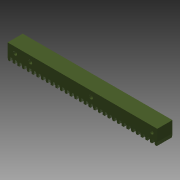
# Autodesk Inventor part: rack
Saved by Autodesk Inventor 2015 (Build 190159000, 159)
## iProperties
Created: 2015-01-14
Part Number: rack
Material: Nylon, molybdenum disulphide
Document SubType Name: Modeling
Designer: Jarod
Density: 1.13 g/cm^3
Appearance: Nylon 6
Author: Jarod
Autodesk Inventor part; units mm, degrees
ref_plane "YZ Plane" through (0, 0, 0) normal (1, 0, 0) x (0, 1, 0)
ref_plane "XZ Plane" through (0, 0, 0) normal (0, 1, 0) x (-1, 0, 0)
ref_plane "XY Plane" through (0, 0, 0) normal (0, 0, 1) x (1, 0, 0)
sketch "Sketch1" plane through (0, 0, 0) normal (1, 0, 0) x (0, 1, 0)
  line L0 (0, 0) -> (25.4, 0)
  line L1 (25.4, 0) -> (25.4, -25.4)
  line L2 (25.4, -25.4) -> (0, -25.4)
  line L3 (0, -25.4) -> (0, 0)
  dimension "d0" = 25.4
  dimension "d1" = 25.4
  constraints: 8 end point, 2 parallel, 1 horizontal, 1 perpendicular
  measures "d0" distance of L1.end L2.end
  measures "d1" distance of L0.end L1.end
extrude "Extrusion1" add sketch "Sketch1" along normal blind 254
sketch "Sketch2" plane through (0, 0, 0) normal (0, 0, 1) x (1, 0, 0)
  line L0 (0, 0) -> (0, 25.4) projected
  line L1 (0, 0) -> (254, 0) projected
  line L2 (254, 25.4) -> (254, 0) projected
  line L3 (0, 25.4) -> (254, 25.4) projected
  line L4 (0, 0) -> (0.7938, 0) construction
  line L5 (0.7938, 0) -> (0.7937, 6.35) construction
  line L6 (0.7937, 6.35) -> (0, 6.35) construction
  line L7 (0, 6.35) -> (0, 0) construction
  line L8 (0.7937, 6.35) -> (3.9687, 6.35) construction
  line L9 (3.9687, 6.35) -> (3.9687, 0) construction
  line L10 (3.9687, 0) -> (0.7938, 0) construction
  line L11 (0.7938, 0) -> (0.7937, 6.35) construction
  line L12 (3.9687, 6.35) -> (4.7625, 6.35) construction
  line L13 (4.7625, 6.35) -> (4.7625, 0) construction
  line L14 (4.7625, 0) -> (3.9687, 0) construction
  line L15 (3.9687, 0) -> (3.9687, 6.35) construction
  line L16 (0, 6.35) -> (0.7938, 0)
  line L17 (0.7938, 0) -> (3.9687, 0)
  line L18 (4.7625, 6.35) -> (7.9375, 6.35) construction
  line L19 (7.9375, 6.35) -> (7.9375, 0) construction
  line L20 (7.9375, 0) -> (4.7625, 0) construction
  line L21 (4.7625, 0) -> (4.7625, 6.35) construction
  line L22 (3.9687, 0) -> (4.7625, 6.35)
  line L23 (4.7625, 6.35) -> (7.9375, 6.35)
  line L24 (7.9375, 6.35) -> (7.9375, 0)
  line L25 (0, 6.35) -> (0, 0)
  line L26 (0, 0) -> (0.7938, 0)
  line L27 (3.9687, 0) -> (7.9375, 0)
  dimension "d4" = 0.7937
  dimension "d5" = 6.35
  dimension "d6" = 3.175
  dimension "d7" = 6.35
  dimension "d8" = 0.7937
  dimension "d9" = 6.35
  dimension "d10" = 3.175
  dimension "d11" = 6.35
  constraints: 48 end point, 11 equal length, 4 horizontal, 4 perpendicular
  measures "d4" distance of L6.end L5.end
  measures "d5" distance of L5.end L4.end
  measures "d6" distance of L9.end L10.end
  measures "d7" distance of L8.end L9.end
  measures "d8" distance of L13.end L14.end
  measures "d9" distance of L12.end L13.end
  measures "d10" distance of L19.end L20.end
  measures "d11" distance of L18.end L19.end
extrude "Extrusion3" cut sketch "Sketch2" against normal blind 25.4 contours L0 L16 L1 | L22 L23 L24 L1
pattern_linear "Rectangular Pattern2" count 32 spacing 7.9375 along (1, 0, 0) of "Extrusion3"
sketch "Sketch4" plane through (0, 25.4, 0) normal (0, 0, 1) x (1, 0, 0)
  line L0 (254, 0) -> (254, -25.4) projected
  line L1 (0, 0) -> (254, 0) projected
  line L2 (0, -19.05) -> (0, 0) projected
  point P0 (0, -25.4)
  point P1 (241.3, -9.525)
  point P2 (12.7, -9.525)
  point P3 (38.1, -9.525)
  point P4 (139.7, -9.525)
  dimension "d33" = 12.7
  dimension "d34" = 9.525
  dimension "d35" = 9.525
  dimension "d44" = 12.7
  dimension "d45" = 38.1
  dimension "d46" = 114.3
  dimension "d47" = 9.525
  dimension "d48" = 9.525
  measures "d33" distance from line of L0 point (241.3, -9.525)
  measures "d34" distance from line of L1 point (241.3, -9.525)
  measures "d35" distance from line of point (12.7, -9.525) L1
  measures "d44" distance from line of L2 point (12.7, -9.525)
  measures "d45" distance from line of L2 point (38.1, -9.525)
  measures "d46" distance from line of L0 point (139.7, -9.525)
  measures "d47" distance from line of L1 point (38.1, -9.525)
  measures "d48" distance from line of L1 point (139.7, -9.525)
hole "Hole3" at (241.3, 15.875, 0) at (12.7, 15.875, 0) at (38.1, 15.875, 0) at (139.7, 15.875, 0) direction (0, 0, -1) diameter 6.35 end through all
sketch "Sketch5" plane through (254, 0, 0) normal (1, 0, 0) x (0, 0, -1)
  line L0 (0, 6.35) -> (25.4, 6.35) projected
  line L1 (25.4, 6.35) -> (25.4, 25.4) projected
  line L2 (25.4, 25.4) -> (0, 25.4) projected
  line L3 (0, 25.4) -> (0, 6.35) projected
  point P0 (0, 0)
extrude "Extrusion4" cut sketch "Sketch5" against normal blind 3.175
body "Solid1"
